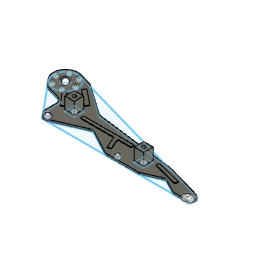
TrackMediumDesign v1 v2 (Autodesk Fusion 360 design; units mm, degrees)
Autodesk Fusion 360 part; units mm, degrees
note: some values were not read from the file. Set by a fixed rule: which sketch regions a step uses.
sketch "Sketch1" plane through (0, 0, 0) normal (0, 0, 1) x (1, 0, 0)
  line L0 (-50.6234, 49.3431) -> (-3.198, -7.4541)
  line L1 (-2.0113, -7.5) -> (224.0597, -7.5)
  line L2 (-30.2635, 80.5455) -> (225.8084, 7.442)
  line L3 (218.275, -2.7029) -> (218.4394, -2.7498)
  arc A0 (225, -2.55) -> (225, 2.55) centre (225, 0) ccw
  arc A1 (224.0597, -7.5) -> (225.8084, 7.442) centre (224.0646, 0.0728) ccw
  arc A2 (-3.198, -7.4541) -> (-2.0113, -7.5) centre (-2.3159, -0.0062) ccw
  arc A3 (-30.2635, 80.5455) -> (-50.6234, 49.3431) centre (-35.6165, 61.7946) ccw
  circle A4 centre (-35.6165, 61.7946) radius 19.5
  line L4 (55, 15) -> (4.1872, -7.5)
  line L5 (-9.5564, 74.634) -> (40, 40)
  line L6 (-10.2571, 1) -> (-10.2571, 29.4154)
  line L7 (-10.2571, 29.4154) -> (-41.41, 38.3089)
  circle A5 centre (220, 0) radius 2.65
  circle A6 centre (-2.3159, -0.0062) radius 2.65
  circle A7 centre (-35.6165, 61.7946) radius 6.25
  circle A8 centre (-35.6165, 61.7946) radius 18.5
  line L8 (5, 35) -> (20, 35)
  line L9 (20, 35) -> (20, 20)
  line L10 (20, 20) -> (5, 20)
  line L11 (5, 20) -> (5, 35)
  line L12 (130, 20) -> (145, 20)
  line L13 (145, 20) -> (145, 5)
  line L14 (145, 5) -> (130, 5)
  line L15 (130, 5) -> (130, 20)
  circle A9 centre (-20.1665, 61.7946) radius 1.55
  circle A10 centre (-27.8915, 75.1747) radius 1.55
  circle A11 centre (-43.3415, 75.1747) radius 1.55
  circle A12 centre (-51.0665, 61.7946) radius 1.55
  circle A13 centre (-43.3415, 48.4145) radius 1.55
  circle A14 centre (-27.8915, 48.4145) radius 1.55
  circle A15 centre (108.8421, -0.0031) radius 2.65
  line L16 (97.1136, -7.5) -> (55, 15)
  line L17 (150.0703, -7.5) -> (179.7021, 5.621)
  line L18 (179.7021, 5.621) -> (204.2609, -7.5)
  line L19 (40, 40) -> (170.5146, 23.2273)
  circle A16 centre (12.5, 27.5) radius 2.65
  circle A17 centre (137.5, 12.5) radius 2.65
  dimension "d10" = 5.1
  dimension "d44" = 39
  dimension "d49" = 5.3
  dimension "d50" = 5.3
  dimension "d66" = 12.5
  dimension "d67" = 37
  dimension "d114" = 3.1
  dimension "d116" = 360
  dimension "d135" = 5.3
  dimension "d140" = 5.3
  dimension "d141" = 5.3
  constraint horizontal L1
  constraint parallel L2 L3
  constraint concentric A3 A4
  constraint coincident L1 L4.end
  constraint coincident L2 L5.start
  constraint coincident L0 L6.start
  constraint coincident L0 L7.end
  constraint parallel L2 L7
  constraint concentric A2 A6
  constraint concentric A4 A7
  constraint concentric A3 A8
  constraint horizontal L8
  constraint vertical L9
  constraint horizontal L10
  constraint vertical L11
  constraint horizontal L12
  constraint vertical L13
  constraint horizontal L14
  constraint vertical L15
  constraint vertical L6
  constraint coincident L1 L16.start
  constraint coincident L1 L17.start
  constraint parallel L4 L17
  constraint coincident L1 L18.end
  constraint parallel L16 L18
  constraint coincident L2 L19.end
  measures "d10" distance of A0.end A0.start
  measures "d44" diameter of A4
  measures "d49" diameter of A5
  measures "d50" diameter of A6
  measures "d66" diameter of A7
  measures "d67" diameter of A8
  measures "d114" diameter of A9
  measures "d135" diameter of A15
  measures "d140" diameter of A16
  measures "d141" diameter of A17
extrude "Extrude24" add sketch "Sketch1" along normal blind 3 contours L0 L1 L2 A1 A2 A4 L4 L5 L6 L7 L16 L17 L18 L19 | A3 A4 | A8 | L8 L9 L10 L11 | L12 L13 L14 L15 | A16 | A17
extrude "Extrude25" add sketch "Sketch1" along normal blind 21.5 contours L8 L9 L10 L11 | L12 L13 L14 L15 | A16 | A17
extrude "Extrude26" cut sketch "Sketch1" along normal blind 22 contours A16 | A17
fillet "Fillet14" radius 5 1 edges at (-41.41, 38.3089, 1.5)
fillet "Fillet15" radius 10 1 edges at (-10.2571, 29.4154, 1.5)
fillet "Fillet16" radius 5 1 edges at (-10.2571, 1, 1.5)
fillet "Fillet17" radius 10 1 edges at (55, 15, 1.5)
fillet "Fillet18" radius 5 1 edges at (97.1136, -7.5, 1.5)
fillet "Fillet19" radius 5 1 edges at (150.0703, -7.5, 1.5)
fillet "Fillet20" radius 10 1 edges at (179.7021, 5.621, 1.5)
fillet "Fillet21" radius 5 1 edges at (204.2609, -7.5, 1.5)
fillet "Fillet22" radius 10 1 edges at (170.5146, 23.2273, 1.5)
fillet "Fillet23" radius 10 1 edges at (40, 40, 1.5)
fillet "Fillet24" radius 5 1 edges at (-9.5564, 74.634, 1.5)
sketch "Sketch4" plane through (0, 0, 3) normal (0, 0, 1) x (-1, 0, 0)
  arc A0 (8.87, -74.1543) -> (10.3617, -74.8639) centre (11.7343, -70.056) ccw
  line L0 (10.3617, -74.8639) -> (30.2635, -80.5455)
  arc A1 (30.2635, -80.5455) -> (50.6234, -49.3431) centre (35.6165, -61.7946) ccw
  line L1 (50.6234, -49.3431) -> (42.396, -39.4898)
  arc A2 (42.396, -39.4898) -> (39.9306, -37.8866) centre (38.558, -42.6945) ccw
  line L2 (39.9306, -37.8866) -> (17.512, -31.4865)
  arc A3 (10.2571, -21.8707) -> (17.512, -31.4865) centre (20.2571, -21.8707) ccw
  line L3 (10.2571, -21.8707) -> (10.2571, -2.813)
  arc A4 (10.2571, -2.813) -> (9.0951, 0.3917) centre (5.2571, -2.813) ccw
  line L4 (9.0951, 0.3917) -> (3.198, 7.4541)
  arc A5 (3.198, 7.4541) -> (2.0113, 7.5) centre (2.3159, 0.0062) ccw
  line L5 (2.0113, 7.5) -> (-4.1872, 7.5)
  line L6 (-4.1872, 7.5) -> (-50.5405, -13.0253)
  arc A6 (-59.3017, -12.7018) -> (-50.5405, -13.0253) centre (-54.5894, -3.8817) ccw
  line L7 (-59.3017, -12.7018) -> (-96.0094, 6.91)
  arc A7 (-96.0094, 6.91) -> (-98.3655, 7.5) centre (-98.3655, 2.5) ccw
  line L8 (-98.3655, 7.5) -> (-149.0128, 7.5)
  arc A8 (-149.0128, 7.5) -> (-151.0373, 7.0718) centre (-149.0128, 2.5) ccw
  line L9 (-151.0373, 7.0718) -> (-175.2426, -3.6463)
  arc A9 (-184.0038, -3.3228) -> (-175.2426, -3.6463) centre (-179.2915, 5.4973) ccw
  line L10 (-184.0038, -3.3228) -> (-203.1567, 6.91)
  arc A10 (-203.1567, 6.91) -> (-205.5128, 7.5) centre (-205.5128, 2.5) ccw
  line L11 (-205.5128, 7.5) -> (-224.0597, 7.5)
  arc A11 (-224.0597, 7.5) -> (-225.8084, -7.442) centre (-224.0646, -0.0728) ccw
  line L12 (-225.8084, -7.442) -> (-171.2385, -23.0206)
  arc A12 (-171.2385, -23.0206) -> (-169.768, -23.3232) centre (-168.4934, -13.4048) ccw
  line L13 (-169.768, -23.3232) -> (-42.4386, -39.6866)
  arc A13 (-37.9848, -41.4084) -> (-42.4386, -39.6866) centre (-43.7132, -49.605) ccw
  line L14 (-37.9848, -41.4084) -> (8.87, -74.1543)
  line L15 (-5, -20) -> (-5, -35)
  line L16 (-5, -35) -> (-20, -35)
  line L17 (-20, -35) -> (-20, -20)
  line L18 (-20, -20) -> (-5, -20)
  line L19 (-130, -5) -> (-130, -20)
  line L20 (-130, -20) -> (-145, -20)
  line L21 (-145, -20) -> (-145, -5)
  line L22 (-145, -5) -> (-130, -5)
  circle A14 centre (35.6165, -61.7946) radius 6.25
  circle A15 centre (2.3159, 0.0062) radius 2.65
  circle A16 centre (20.1665, -61.7946) radius 1.55
  circle A17 centre (43.3415, -48.4145) radius 1.55
  circle A18 centre (27.8915, -75.1747) radius 1.55
  circle A19 centre (43.3415, -75.1747) radius 1.55
  circle A20 centre (51.0665, -61.7946) radius 1.55
  circle A21 centre (-220, 0) radius 2.65
  circle A22 centre (27.8915, -48.4145) radius 1.55
  circle A23 centre (-108.8421, 0.0031) radius 2.65
  line L23 (-155, -20) -> (-195, -10)
  line L24 (-195, -10) -> (-193.7855, -5.142)
  line L25 (-193.7855, -5.142) -> (-154.3536, -15)
  line L26 (-154.3536, -15) -> (-155, -20)
  line L27 (-30, -25) -> (-110, -25)
  line L28 (-110, -25) -> (-110, -20)
  line L29 (-110, -20) -> (-30, -20)
  line L30 (-30, -20) -> (-30, -25)
  line L31 (-85, -15) -> (-91.3581, -0.6413)
  line L32 (-91.3581, -0.6413) -> (-96.149, -2.7627)
  line L33 (-96.149, -2.7627) -> (-90.238, -16.1118)
  line L34 (-90.238, -16.1118) -> (-89.4127, -20)
  line L35 (-85, -15) -> (-82.786, -20)
  line L36 (5, -65) -> (-20, -44.6537)
  line L37 (-20, -44.6537) -> (-16.1568, -39.9315)
  line L38 (-16.1568, -39.9315) -> (8.0754, -59.653)
  line L39 (8.0754, -59.653) -> (5, -65)
  line L40 (21.4667, -42.2926) -> (3.0133, -20.8693)
  line L41 (3.0133, -20.8693) -> (-1.2182, -24.5142)
  line L42 (-1.2182, -24.5142) -> (16.473, -45.0526)
  line L43 (16.473, -45.0526) -> (21.4667, -42.2926)
  constraint perpendicular L23 L24
  constraint perpendicular L24 L25
  constraint horizontal L27
  constraint perpendicular L27 L28
  constraint perpendicular L28 L29
  constraint perpendicular L27 L30
  constraint perpendicular L6 L31
  constraint perpendicular L31 L32
  constraint perpendicular L32 L33
  constraint coincident L29 L34.end
  constraint coincident L29 L35.end
  constraint parallel L31 L35
  constraint perpendicular L36 L37
  constraint perpendicular L37 L38
  constraint perpendicular L40 L41
  constraint perpendicular L41 L42
extrude "Extrude27" add sketch "Sketch4" along normal blind 1 contours L23 L24 L25 L26 | L27 L28 L29 L30 | L29 L31 L32 L33 L34 L35 | L36 L37 L38 L39 | L40 L41 L42 L43
